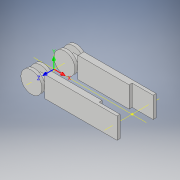
# Autodesk Inventor part: link_2
Saved by Autodesk Inventor 2019 (Build 230136000, 136)
## iProperties
Created: 2020-08-30
Part Number: link_2
Material: Generic
Document SubType Name: Modeling
Designer: Daniel
Density: 1 g/cm^3
Appearance: Default
Author: Daniel
Autodesk Inventor part; units mm, degrees
ref_plane "YZ Plane" through (0, 0, 0) normal (1, 0, 0) x (0, 1, 0)
ref_plane "Work Plane1" through (0, 0, 28) normal (0, 0, 1) x (1, 0, 0)
sketch "Sketch2" plane through (0, 0, 28) normal (0, 0, 1) x (1, 0, 0)
  circle A0 centre (0, 0) radius 28
  dimension "d2" = 56
  constraints: 1 centre point, 1 coincident
  measures "d2" diameter of A0
extrude "Extrusion1" add sketch "Sketch2" along normal blind 8
sketch "Sketch3" plane through (0, 0, 36) normal (0, 0, 1) x (1, 0, 0)
  line L0 (28, -12) -> (0, -12)
  line L1 (0, -12) -> (0, 12)
  line L2 (0, 12) -> (28, 12)
  line L3 (28, 12) -> (28, -12)
  line L4 (28, -12) -> (0, 12) construction
  line L5 (0, -12) -> (28, 12) construction
  line L6 (-77.6, 0) -> (269.6, 0) projected
  line L7 (28, -28) -> (220, -28)
  line L8 (220, -28) -> (220, 28)
  line L9 (220, 28) -> (28, 28)
  line L10 (28, 28) -> (28, -28)
  line L11 (28, -28) -> (220, 28) construction
  line L12 (220, -28) -> (28, 28) construction
  point P0 (0, 0)
  point P1 (14, 0)
  point P2 (124, 0)
  dimension "d5" = 24
  dimension "d6" = 28
  dimension "d7" = 192
  dimension "d8" = 56
  constraints: 24 end point, 5 midpoint, 4 parallel, 2 horizontal, 2 perpendicular, 2 point on line, 1 collinear
  measures "d5" distance between parallel lines of L0 L2
  measures "d6" distance between parallel lines of L3 L1
  measures "d7" distance of L8.end L9.end
  measures "d8" distance between parallel lines of L7 L9
extrude "Extrusion2" add sketch "Sketch3" along normal blind 16
sketch "Sketch4" plane through (0, 0, 52) normal (0, 0, 1) x (1, 0, 0)
  circle A0 centre (0, 0) radius 28
  arc A1 (25.2982, 12) -> (25.2982, -12) centre (0, 0) ccw projected
  constraints: 1 centre point, 1 coincident, 1 concentric
extrude "Extrusion3" add sketch "Sketch4" along normal blind 8
sketch "Sketch5" plane through (0, 0, 36) normal (0, 0, -1) x (-1, 0, 0)
  line L0 (-28, -28) -> (-220, -28) projected
  line L1 (-220, 28) -> (-28, 28) projected
  line L2 (-220, -28) -> (-164, -28)
  line L3 (-164, -28) -> (-164, 28)
  line L4 (-164, 28) -> (-220, 28)
  line L5 (-220, 28) -> (-220, -28)
  line L6 (77.6, 0) -> (-269.6, 0) projected
  point P0 (0, 0)
  point P1 (-208, 0)
  dimension "d13" = 56
  dimension "d16" = 12
  constraints: 8 end point, 2 parallel, 2 point on line, 1 horizontal, 1 perpendicular
  measures "d13" distance between parallel lines of L3 L5
  measures "d16" distance from line of L5 point (-208, 0)
extrude "Extrusion4" cut sketch "Sketch5" against normal blind 8
mirror "Mirror2" about plane through (0, 0, 0) normal (0, 0, 1) of "Extrusion1", "Extrusion2", "Extrusion3", "Extrusion4"
ref_plane "Work Plane3" through (0, 28, 0) normal (0, 1, 0) x (-1, 0, 0)
ref_plane "UCS2: YZ Plane" through (0, 0, 0) normal (1, 0, 0) x (0, 1, 0)
ref_plane "UCS2: XZ Plane" through (0, 0, 0) normal (0, 1, 0) x (0, 0, 1)
ref_plane "UCS2: XY Plane" through (0, 0, 0) normal (0, 0, 1) x (1, 0, 0)
body "Solid1"
